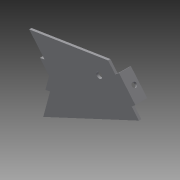
# Autodesk Inventor part: Right Bicep
Saved by Autodesk Inventor 2014 SP2 (Build 180246200, 246)
## iProperties
Created: 2015-08-01
Part Number: Right Bicep
Material: Generic
Document SubType Name: Modeling
Designer: Devon
Density: 1 g/cm^3
Appearance: Default
Author: Devon
Autodesk Inventor part; units mm, degrees
ref_plane "YZ Plane" through (0, 0, 0) normal (1, 0, 0) x (0, 1, 0)
ref_plane "XZ Plane" through (0, 0, 0) normal (0, 1, 0) x (-1, 0, 0)
ref_plane "XY Plane" through (0, 0, 0) normal (0, 0, 1) x (1, 0, 0)
sketch "Sketch1" plane through (0, 0, 0) normal (0, 0, 1) x (1, 0, 0)
  line L0 (-10.4788, 3.5567) -> (22.1748, -35.3584)
  line L1 (-10.4788, 3.5567) -> (40.3212, 3.5567) construction
  line L2 (22.1748, -35.3584) -> (8.205, -87.4942)
  line L3 (8.205, -87.4942) -> (134.8162, -28.4545)
  line L4 (134.8162, -28.4545) -> (93.9992, 20.1894)
  line L5 (93.9992, 20.1894) -> (-10.4788, 3.5567)
  point P0 (0, 0)
  dimension "d0" = 50.8
  dimension "d1" = 50
  dimension "d2" = 53.975
  dimension "d3" = 125
  dimension "d4" = 139.7
  dimension "d5" = 50
  dimension "d6" = 63.5
  dimension "d7" = 75
  constraints: 12 end point, 1 equal length, 1 horizontal, 1 parallel
  measures "d0" distance of L0.start L0.end
  measures "d1" angle of L0 L1
  measures "d2" distance of L0.end L2.end
  measures "d3" angle of L0 L2
  measures "d4" distance of L2.end L3.end
  measures "d5" angle of L3 L2
  measures "d6" distance of L3.end L4.end
  measures "d7" angle of L4 L3
extrude "Extrusion1" add sketch "Sketch1" along normal blind 3.175
sketch "Sketch2" plane through (0, 0, 3.175) normal (0, 0, 1) x (1, 0, 0)
  line L0 (-10.4788, 3.5567) -> (22.1748, -35.3584) projected
  line L1 (22.1748, -35.3584) -> (8.205, -87.4942) projected
  line L2 (22.1748, -35.3584) -> (9.9297, -20.7652)
  line L3 (22.1748, -35.3584) -> (17.2443, -53.7593)
  line L4 (9.9297, -20.7652) -> (3.7302, -22.1396)
  line L5 (17.2443, -53.7593) -> (11.0448, -55.1337)
  line L6 (15.9753, -36.7328) -> (3.7302, -22.1396)
  line L7 (15.9753, -36.7328) -> (11.0448, -55.1337)
  point P0 (0, 0)
  dimension "d10" = 19.05
  dimension "d11" = 19.05
  dimension "d12" = 6.35
  dimension "d13" = 6.35
  dimension "d14" = 6.35
  constraints: 12 end point, 2 point on line, 1 parallel
  measures "d10" distance of L0.end L2.end
  measures "d11" distance of L0.end L3.end
  measures "d12" distance of L2.end L4.end
  measures "d13" distance of L3.end L5.end
  measures "d14" distance of L0.end L6.start
extrude "Extrusion2" add sketch "Sketch2" against normal blind 3.175
sketch "Sketch3" plane through (0, 0, 0) normal (0, 0, -1) x (-1, 0, 0)
  line L0 (-17.2443, -53.7593) -> (-11.0448, -55.1337) projected
  line L1 (-11.0448, -55.1337) -> (-15.9753, -36.7328) projected
  line L2 (-15.9753, -36.7328) -> (-3.7302, -22.1396) projected
  line L3 (-3.7302, -22.1396) -> (-9.9297, -20.7652) projected
  line L4 (-3.7302, -22.1396) -> (-6.83, -21.4524)
  line L5 (-11.0448, -55.1337) -> (-14.1446, -54.4465)
  line L6 (-14.1446, -54.4465) -> (-19.0751, -36.0456)
  line L7 (-6.83, -21.4524) -> (-19.0751, -36.0456)
  point P0 (0, 0)
  dimension "d17" = 3.175
  dimension "d18" = 3.175
  constraints: 8 end point, 2 midpoint, 2 parallel
  measures "d17" distance of L2.end L4.end
  measures "d18" distance of L0.end L5.end
extrude "Extrusion3" add sketch "Sketch3" along normal blind 12.7
sketch "Sketch4" plane through (3.7302, -22.1396, -12.7) normal (-0.7660444, -0.6427876, 0) x (0, 0, 1)
  line L0 (0, -19.05) -> (0, 0) projected
  line L1 (15.875, -19.05) -> (0, -19.05) projected
  line L2 (0, -9.525) -> (6.35, -9.525)
  point P0 (12.7, 19.3577)
  dimension "d21" = 6.35
  constraints: 2 end point, 1 midpoint, 1 parallel
  measures "d21" distance of L2.start L2.end
hole "Hole1" at (9.8528, -29.4362, -6.35) direction (0.7660444, 0.6427876, 0) diameter 6.35 end through all
sketch "Sketch5" plane through (15.9753, -36.7328, -12.7) normal (-0.9659258, 0.258819, 0) x (0, 0, 1)
  line L0 (0, -19.05) -> (0, 0) projected
  line L1 (15.875, -19.05) -> (0, -19.05) projected
  line L2 (0, -9.525) -> (6.35, -9.525)
  point P0 (12.7, 31.3464)
  dimension "d29" = 6.35
  constraints: 2 end point, 1 midpoint, 1 parallel
  measures "d29" distance of L2.start L2.end
hole "Hole2" at (13.5101, -45.9332, -6.35) direction (0.9659258, -0.258819, 0) diameter 6.35 end through all
sketch "Sketch6" plane through (0, 0, 0) normal (0, 0, -1) x (-1, 0, 0)
  line L0 (-134.8162, -28.4545) -> (-93.9992, 20.1894) projected
  line L1 (-114.4077, -4.1326) -> (-103.5422, 8.8164)
  line L2 (-114.4077, -4.1326) -> (-125.2732, -17.0815)
  line L3 (-125.2732, -17.0815) -> (-130.1376, -12.9998)
  line L4 (-130.1376, -12.9998) -> (-108.4066, 12.8981)
  line L5 (-108.4066, 12.8981) -> (-103.5422, 8.8164)
  point P0 (0, 0)
  dimension "d37" = 16.9037
  dimension "d38" = 16.9037
  dimension "d39" = 6.35
  dimension "d40" = 33.8074
  constraints: 10 end point, 2 point on line, 1 midpoint, 1 parallel, 1 perpendicular
  measures "d37" distance of L1.start L1.end
  measures "d38" distance of L1.start L2.end
  measures "d39" distance of L2.end L3.end
  measures "d40" distance of L3.end L4.end
extrude "Extrusion4" add sketch "Sketch6" against normal blind 3.175
sketch "Sketch7" plane through (0, 0, 0) normal (0, 0, -1) x (-1, 0, 0)
  line L0 (-103.5422, 8.8164) -> (-108.4066, 12.8981) projected
  line L1 (-108.4066, 12.8981) -> (-130.1376, -12.9998) projected
  line L2 (-130.1376, -12.9998) -> (-125.2732, -17.0815) projected
  line L3 (-108.4066, 12.8981) -> (-130.1376, -12.9998)
  line L4 (-130.1376, -12.9998) -> (-127.7054, -15.0407)
  line L5 (-127.7054, -15.0407) -> (-105.9744, 10.8573)
  line L6 (-105.9744, 10.8573) -> (-108.4066, 12.8981)
  point P0 (0, 0)
  dimension "d43" = 3.175
  constraints: 8 end point, 2 collinear, 2 midpoint
  measures "d43" distance of L1.end L4.end
extrude "Extrusion5" add sketch "Sketch7" along normal blind 12.7
sketch "Sketch8" plane through (108.4066, 12.8981, 3.175) normal (0.7660444, 0.6427876, 0) x (0, 0, -1)
  line L0 (15.875, 0) -> (15.875, -33.8074) projected
  line L1 (15.875, -16.9037) -> (9.525, -16.9037)
  point P0 (3.175, 59.8019)
  dimension "d46" = 6.35
  constraints: 2 end point, 1 midpoint, 1 perpendicular
  measures "d46" distance of L1.start L1.end
hole "Hole3" at (119.2721, -0.0509, -6.35) direction (-0.7660444, -0.6427876, 0) diameter 6.35 end through all
sketch "Sketch9" plane through (0, 0, 3.175) normal (0, 0, 1) x (1, 0, 0)
  line L0 (130.1376, -12.9998) -> (108.4066, 12.8981) projected
  line L1 (103.5422, 8.8164) -> (93.9992, 20.1894) projected
  line L2 (93.9992, 20.1894) -> (-10.4788, 3.5567) projected
  line L3 (71.6563, 16.6324) -> (76.7318, -15.2495)
  line L4 (111.0345, 9.7664) -> (80.0581, -16.2259)
  line L5 (80.0581, -16.2259) -> (74.7441, -9.893)
  line L6 (76.7318, -15.2495) -> (78.9434, -14.8974)
  line L7 (17.2443, -53.7593) -> (8.205, -87.4942) projected
  line L8 (11.0448, -55.1337) -> (34.2557, 31.4904)
  line L9 (78.9434, -14.8974) -> (25.6522, -0.6181)
  line L10 (78.9434, -14.8974) -> (82.2304, -2.6302)
  point P0 (0, 0)
  dimension "d54" = 32.2834
  dimension "d55" = 40.4368
  dimension "d71" = 12.7
  constraints: 14 end point, 6 perpendicular, 4 point on line, 1 parallel
  measures "d54" distance of L3.start L3.end
  measures "d55" distance of L4.start L4.end
  measures "d71" distance of L6.end L10.end
hole "Hole6" at (82.2304, -2.6302, 3.175) direction (0, 0, -1) diameter 7.9375 end through all
body "Solid1"
